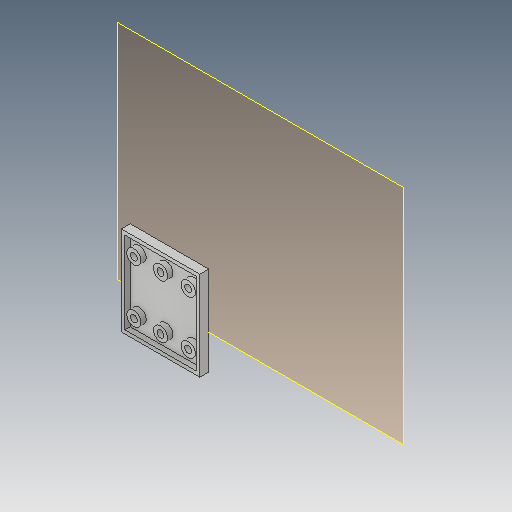
# Autodesk Inventor part: 02_Zeiss_Axiotech_adapterplate_rightleft_connector
Saved by Autodesk Inventor 2019 (Build 230136000, 136)
## iProperties
Created: 2019-05-07
Part Number: 02_Zeiss_Axiotech_adapterplate_rightleft_connector
Material: Generic
Document SubType Name: Modeling
Designer: diederichbenedict
Density: 1 g/cm^3
Appearance: Default
Author: diederichbenedict
Autodesk Inventor part; units mm, degrees
ref_plane "YZ Plane" through (0, 0, 0) normal (1, 0, 0) x (0, 1, 0)
ref_plane "XZ Plane" through (0, 0, 0) normal (0, 1, 0) x (-1, 0, 0)
ref_plane "XY Plane" through (0, 0, 0) normal (0, 0, 1) x (1, 0, 0)
ref_plane "Work Plane1" through (0, 0, 0) normal (0, 0, 1) x (1, 0, 0)
sketch "Sketch1" plane through (0, 0, 0) normal (0, 0, 1) x (1, 0, 0)
  circle A0 centre (-66, -92.5) radius 1.95 projected
  circle A1 centre (-51, -92.5) radius 1.95 projected
  circle A2 centre (-35.4846, -92.6897) radius 1.95 projected
  circle A3 centre (-35.4846, -122.3103) radius 1.95 projected
  circle A4 centre (-51, -122.5) radius 1.95 projected
  circle A5 centre (-66, -122.5) radius 1.95 projected
  line L0 (-26, -87.5) -> (-26, -107.5) construction
  line L1 (-21, -87.5) -> (-26, -87.5) construction
  line L2 (-21, -87.5) -> (-21, -6) construction
  line L3 (-21, -6) -> (73, -6) construction
  line L4 (73, -6) -> (73, 6) construction
  line L5 (73, 6) -> (-73, 6) construction
  line L6 (-73, 6) -> (-73, -107.5) construction
  line L7 (-73, -107.5) -> (-26, -107.5) construction
  circle A6 centre (-51, -92.5) radius 1.95 construction
  circle A7 centre (-26, -72.5) radius 1.95 construction
  circle A8 centre (-51, -22.5) radius 1.95 construction
  circle A9 centre (-26, -22.5) radius 1.95 construction
  circle A10 centre (67, 0) radius 1.95 construction
  circle A11 centre (-67, 0) radius 1.95 construction
  circle A12 centre (-26, -47.5) radius 1.95 construction
  circle A13 centre (-51, -72.5) radius 1.95 construction
  circle A14 centre (-35.4846, -92.6897) radius 1.95 construction
  circle A15 centre (-66, -92.5) radius 1.95 construction
  circle A16 centre (-51, -47.5) radius 19.7399 construction
  line L8 (-26, -127.5) -> (-26, -107.5) construction
  line L9 (-73, -107.5) -> (-26, -107.5) construction
  line L10 (-73, -221) -> (-73, -107.5) construction
  line L11 (73, -221) -> (-73, -221) construction
  line L12 (73, -209) -> (73, -221) construction
  line L13 (-21, -209) -> (73, -209) construction
  line L14 (-21, -127.5) -> (-21, -209) construction
  line L15 (-21, -127.5) -> (-26, -127.5) construction
  circle A17 centre (-51, -122.5) radius 1.95 construction
  circle A18 centre (-26, -142.5) radius 1.95 construction
  circle A19 centre (-51, -192.5) radius 1.95 construction
  circle A20 centre (-26, -192.5) radius 1.95 construction
  circle A21 centre (67, -215) radius 1.95 construction
  circle A22 centre (-67, -215) radius 1.95 construction
  circle A23 centre (-26, -167.5) radius 1.95 construction
  circle A24 centre (-51, -142.5) radius 1.95 construction
  circle A25 centre (-35.4846, -122.3103) radius 1.95 construction
  circle A26 centre (-66, -122.5) radius 1.95 construction
  circle A27 centre (-51, -167.5) radius 19.7399 construction
  line L16 (-29, -132.5) -> (-73, -132.5)
  line L17 (-73, -132.5) -> (-73, -82.5)
  line L18 (-73, -82.5) -> (-29, -82.5)
  line L19 (-29, -82.5) -> (-29, -132.5)
  line L20 (-29, -132.5) -> (-73, -82.5) construction
  line L21 (-73, -132.5) -> (-29, -82.5) construction
  point P0 (0, 0)
  point P1 (-51, -107.5)
  dimension "d0" = 44
  dimension "d1" = 50
  constraints: 12 end point, 2 midpoint, 2 parallel, 1 horizontal, 1 perpendicular, 1 point on line
  measures "d0" distance of L17.end L18.end
  measures "d1" distance of L16.end L17.end
extrude "Extrusion1" add sketch "Sketch1" along normal blind 5
shell "Shell1" thickness 2 removed faces 1 at (-41.1644, -111.8922, 5)
body "Solid1"
